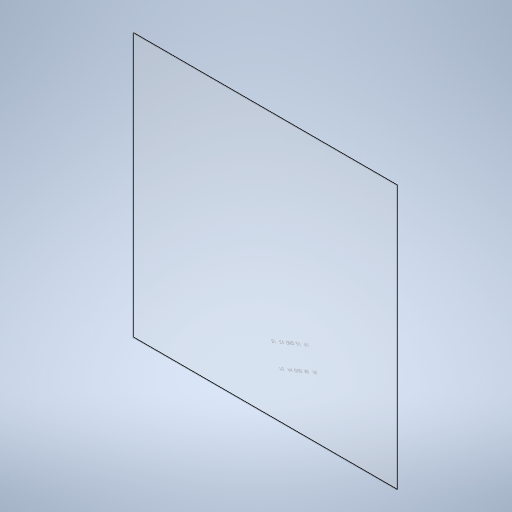
# Autodesk Inventor part: Clippard 8-MC 3D PCB Bottom
Saved by Autodesk Inventor 2024.2 (Build 282272000, 272)
## iProperties
Created: 2024-03-21
Part Number: Clippard 8-MC 3D PCB Bottom
Material: Generic
Document SubType Name: Modeling
Designer: shann
Density: 1 g/cm^3
Appearance: Clear - Light
Author: shann
Autodesk Inventor part; units mm, degrees
ref_plane "YZ Plane" through (0, 0, 0) normal (1, 0, 0) x (0, 1, 0)
ref_plane "XZ Plane" through (0, 0, 0) normal (0, 1, 0) x (-1, 0, 0)
ref_plane "XY Plane" through (0, 0, 0) normal (0, 0, 1) x (1, 0, 0)
sketch "Sketch1" plane through (0, 0, 0) normal (0, 0, 1) x (1, 0, 0)
  line L0 (0, 0) -> (75.184, 0)
  line L1 (75.184, 0) -> (75.184, -75.184)
  line L2 (75.184, -75.184) -> (0, -75.184)
  line L3 (0, -75.184) -> (0, 0)
  dimension "d5" = 75.184
  constraints: 1 coincident, 1 horizontal, 2 other
  measures "d5" distance of L2.end L0.start
extrude "Extrusion1" add sketch "Sketch1" along normal blind 0.254
body "Solid1"
